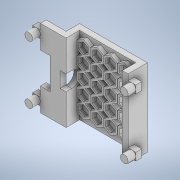
# Autodesk Inventor part: f2_grip
Saved by Autodesk Inventor 2020 (Build 240168000, 168)
## iProperties
Created: 2019-10-20
Part Number: f2_grip
Material: Generic
Document SubType Name: Modeling
Designer: ayad493
Density: 1 g/cm^3
Appearance: Default
Author: ayad493
Autodesk Inventor part; units mm, degrees
ref_plane "YZ Plane" through (0, 0, 0) normal (1, 0, 0) x (0, 1, 0)
ref_plane "XZ Plane" through (0, 0, 0) normal (0, 1, 0) x (-1, 0, 0)
ref_plane "XY Plane" through (0, 0, 0) normal (0, 0, 1) x (1, 0, 0)
sketch "Sketch1" plane through (0, 0, 0) normal (0, 0, 1) x (1, 0, 0)
  line L0 (0, 0) -> (16, 0)
  line L1 (16, 0) -> (16, -20)
  line L2 (16, -20) -> (0, -20)
  line L3 (0, -20) -> (0, 0)
  line L4 (16, 0) -> (14.5, 0)
  line L5 (14.5, 0) -> (14.5, -20)
  line L6 (16, 0) -> (16, -1.5)
  line L7 (16, -1.5) -> (18, -1.5)
  line L8 (18, -1.5) -> (18, -3.5)
  line L9 (18, -3.5) -> (16, -3.5)
  line L10 (16, -3.5) -> (16, -1.5)
  line L11 (16, -20) -> (16, -18.5)
  line L12 (16, -18.5) -> (18, -18.5)
  line L13 (18, -18.5) -> (18, -16.5)
  line L14 (18, -16.5) -> (16, -16.5)
  line L15 (16, -16.5) -> (16, -18.5)
  line L16 (18, -2.5) -> (-8.623, -2.5)
  line L17 (-8.623, -2.5) -> (-8.623, -1.5)
  line L18 (-8.623, -1.5) -> (-6.623, -1.5)
  line L19 (-6.623, -1.5) -> (-6.623, -3.5)
  line L20 (-6.623, -3.5) -> (-8.623, -3.5)
  line L21 (-8.623, -3.5) -> (-8.623, -1.5)
  line L22 (0, 0) -> (-6.623, 0)
  line L23 (-6.623, 0) -> (-6.623, -20)
  line L24 (-6.623, -20) -> (0, -20)
  line L25 (18, -17.5) -> (-6.623, -17.5)
  line L26 (-6.623, -17.5) -> (-6.623, -16.5)
  line L27 (-6.623, -16.5) -> (-8.623, -16.5)
  line L28 (-8.623, -16.5) -> (-8.623, -18.5)
  line L29 (-8.623, -18.5) -> (-6.623, -18.5)
  line L30 (-6.623, -18.5) -> (-6.623, -16.5)
  dimension "d0" = 16
  dimension "d1" = 20
  dimension "d2" = 90
  dimension "d3" = 1.5
  dimension "d4" = 1.5
  dimension "d5" = 2
  dimension "d6" = 2
  dimension "d7" = 1.5
  dimension "d8" = 2
  dimension "d9" = 2
  dimension "d10" = 26.623
  dimension "d11" = 2
  dimension "d12" = 1
  dimension "d13" = 2
  constraints: 62 end point, 9 perpendicular, 8 parallel, 7 horizontal, 7 point on line, 2 midpoint, 1 collinear, 1 vertical
  measures "d0" distance of L0.start L0.end
  measures "d1" distance of L0.end L1.end
  measures "d2" angle of L0 L1
  measures "d3" distance of L0.end L4.end
  measures "d4" distance of L0.end L6.end
  measures "d5" distance of L8.end L9.end
  measures "d6" distance of L7.end L8.end
  measures "d7" distance of L1.end L11.end
  measures "d8" distance of L14.end L13.end
  measures "d9" distance of L12.end L13.end
  measures "d10" distance of L16.start L16.end
  measures "d11" distance of L19.end L20.end
  measures "d12" distance of L25.end L26.end
  measures "d13" distance of L29.end L28.end
extrude "Extrusion1" add sketch "Sketch1" along normal blind 1.5
sketch "Sketch2" plane through (0, 0, 1.5) normal (0, 0, 1) x (1, 0, 0)
  line L0 (-8.623, -1.5) -> (-8.623, -3.5) projected
  line L1 (-8.623, -3.5) -> (-6.623, -3.5) projected
  line L2 (-8.623, -1.5) -> (-6.623, -3.5)
  line L3 (18, -3.5) -> (18, -1.5) projected
  line L4 (16, -16.5) -> (16, -3.5) projected
  line L5 (18, -1.5) -> (16, -3.5)
  line L6 (-6.623, -16.5) -> (-8.623, -16.5) projected
  line L7 (-6.623, -18.5) -> (-6.623, -20) projected
  line L8 (-8.623, -16.5) -> (-6.623, -18.5)
  line L9 (16, -18.5) -> (18, -18.5) projected
  line L10 (18, -16.5) -> (16, -16.5) projected
  line L11 (16, -18.5) -> (18, -16.5)
  circle A0 centre (-7.623, -2.5) radius 1
  circle A1 centre (17, -2.5) radius 1
  circle A2 centre (17, -17.5) radius 1
  circle A3 centre (-7.623, -17.5) radius 1
  point P0 (0, 0)
  constraints: 8 end point, 4 centre point, 4 midpoint
extrude "Extrusion2" add sketch "Sketch2" along normal blind 2 contours A0 L2 | A0 L2 | A1 L5 | A2 L11 | L5 A1 | A2 L11 | A3 L8 | L8 A3
sketch "Sketch3" plane through (0, 0, 0) normal (0, 0, -1) x (-1, 0, 0)
  line L0 (6.623, -18.5) -> (6.623, -20) projected
  line L1 (6.623, -20) -> (0, -20)
  line L2 (0, -20) -> (0, 0)
  line L3 (0, 0) -> (6.623, 0)
  line L4 (6.623, 0) -> (6.623, -20)
  line L5 (6.623, -20) -> (-16, -20) projected
  line L6 (-16, 0) -> (6.623, 0) projected
  line L7 (-16, -20) -> (-14.5, -20)
  line L8 (-14.5, -20) -> (-14.5, 0)
  line L9 (-14.5, 0) -> (-16, 0)
  line L10 (-16, 0) -> (-16, -20)
  line L11 (6.623, -20) -> (-16, -20)
  line L12 (-16, -20) -> (-16, -18.5)
  line L13 (-16, -18.5) -> (6.623, -18.5)
  line L14 (6.623, -18.5) -> (6.623, -20)
  line L15 (-16, 0) -> (6.623, 0)
  line L16 (6.623, 0) -> (6.623, -1.5)
  line L17 (6.623, -1.5) -> (-16, -1.5)
  line L18 (-16, -1.5) -> (-16, 0)
  point P0 (0, -1.5)
  point P1 (0, -18.5)
  point P2 (-14.5, -18.5)
  point P3 (-14.5, -1.5)
  dimension "d18" = 1.5
  constraints: 32 end point, 8 parallel, 4 horizontal, 4 perpendicular, 1 point on line
  measures "d18" distance of L9.end L8.end
extrude "Extrusion3" add sketch "Sketch3" along normal blind 5 contours L13 L2 L17 L4 | L0 L1 L2 L13 | L17 L2 L3 L4 | L2 L5 L8 L13 | L17 L8 L6 L2 | L13 L10 L17 L8 | L8 L5 L10 L13 | L17 L10 L6 L8
sketch "Sketch4" plane through (0, 0, 0) normal (0, 0, -1) x (-1, 0, 0)
  line L0 (-14.5, -18.5) -> (0, -18.5) projected
  line L1 (-14.5, -18.5) -> (-14.5, -1.5) projected
  line L2 (0, -18.5) -> (-14.5, -18.5)
  line L3 (-14.5, -18.5) -> (-14.5, -1.5)
  line L4 (-14.5, -1.5) -> (0, -1.5)
  line L5 (0, -1.5) -> (0, -18.5)
  point P0 (0, 0)
  constraints: 8 end point, 2 parallel, 1 horizontal, 1 perpendicular
extrude "Extrusion4" cut sketch "Sketch4" against normal through all
sketch "Sketch5" plane through (-6.623, 0, 1.5) normal (0, 1, 0) x (1, 0, 0)
  line L0 (22.623, 6.5) -> (22.623, 0) projected
  line L1 (0, 6.5) -> (22.623, 6.5)
  line L2 (22.623, 6.5) -> (22.623, 5)
  line L3 (22.623, 5) -> (0, 5)
  line L4 (0, 5) -> (0, 6.5)
  point P0 (6.623, 1.5)
  dimension "d23" = 1.5
  constraints: 8 end point, 2 parallel, 1 horizontal, 1 perpendicular, 1 point on line
  measures "d23" distance of L1.end L2.end
extrude "Extrusion5" add sketch "Sketch5" against normal up to surface (20 mm away)
sketch "Sketch7" plane through (-6.623, -20, 1.5) normal (0, -1, 0) x (1, 0, 0)
  line L0 (21.123, 0) -> (6.623, 0) projected
  line L1 (22.623, -6.5) -> (0, -6.5) projected
  line L2 (6.623, 0) -> (5.123, 0)
  line L3 (5.123, 0) -> (5.123, -6.5)
  line L4 (5.123, -6.5) -> (6.623, -6.5)
  line L5 (6.623, -6.5) -> (6.623, 0)
  line L6 (0, -6.5) -> (0, 0) projected
  line L7 (5.123, -6.5) -> (0, -6.5)
  line L8 (0, -6.5) -> (0, -1.5)
  line L9 (0, -1.5) -> (5.123, -1.5)
  line L10 (5.123, -1.5) -> (5.123, -6.5)
  point P0 (6.623, -1.5)
  dimension "d31" = 1.5
  constraints: 16 end point, 4 parallel, 2 horizontal, 2 perpendicular, 2 point on line
  measures "d31" distance of L4.end L3.end
extrude "Extrusion7" cut sketch "Sketch7" against normal through all contours L1 L6 L9 L3
sketch "Sketch8" plane through (-6.623, -20, 1.5) normal (0, -1, 0) x (1, 0, 0)
  line L0 (22.623, -6.5) -> (22.623, 0) projected
  line L1 (5.123, -1.5) -> (5.123, -6.5) projected
  line L2 (22.623, -6.5) -> (5.123, -6.5)
  line L3 (5.123, -6.5) -> (5.123, -4.9793)
  line L4 (5.123, -4.9793) -> (22.623, -4.9793)
  line L5 (22.623, -4.9793) -> (22.623, -6.5)
  point P0 (6.623, -1.5)
  constraints: 8 end point, 2 parallel, 1 horizontal, 1 perpendicular, 1 point on line
extrude "Extrusion8" cut sketch "Sketch8" against normal through all
sketch "Sketch9" plane through (-6.623, -20, 1.5) normal (0, -1, 0) x (1, 0, 0)
  line L0 (5.123, -4.9793) -> (22.623, -4.9793) projected
  line L1 (5.123, -1.5) -> (5.123, -4.9793) projected
  line L2 (22.623, -4.9793) -> (5.123, -4.9793)
  line L3 (5.123, -4.9793) -> (5.123, -3.4793)
  line L4 (5.123, -3.4793) -> (22.623, -3.4793)
  line L5 (22.623, -3.4793) -> (22.623, -4.9793)
  point P0 (6.623, -1.5)
  dimension "d36" = 1.5
  constraints: 8 end point, 2 parallel, 1 horizontal, 1 perpendicular, 1 point on line
  measures "d36" distance of L2.end L3.end
extrude "Extrusion9" add sketch "Sketch9" against normal up to surface (20 mm away)
sketch "Sketch10" plane through (-6.623, -16.5, 0) normal (-1, 0, 0) x (0, 0, 1)
  line L0 (0, 13) -> (0, 0) projected
  line L1 (1.5, 0) -> (1.5, 13) projected
  line L2 (0, 6.5) -> (1.5, 6.5)
  line L3 (1.5, 6.5) -> (1.5, 2.5)
  line L4 (1.5, 2.5) -> (0, 2.5)
  line L5 (0, 2.5) -> (0, 6.5)
  line L6 (1.5, 6.5) -> (0, 6.5)
  line L7 (0, 6.5) -> (0, 10.5)
  line L8 (0, 10.5) -> (1.5, 10.5)
  line L9 (1.5, 10.5) -> (1.5, 6.5)
  point P0 (0, 16.5)
  point P1 (0, 2.5)
  dimension "d39" = 4
  dimension "d40" = 4
  constraints: 16 end point, 4 parallel, 2 horizontal, 2 perpendicular, 2 point on line, 1 midpoint
  measures "d39" distance of L2.end L3.end
  measures "d40" distance of L6.end L7.end
extrude "Extrusion10" cut sketch "Sketch10" against normal up to surface (5.123 mm away)
sketch "Sketch12" plane through (0, -18.5, -1.9793) normal (0, 0, 1) x (1, 0, 0)
  line L0 (14.5, 0) -> (0, 0) projected
  line L1 (14.5, 17) -> (14.5, 0) projected
  line L2 (14.5, 0) -> (14.5, 4)
  line L3 (12.5, 0) -> (10.7679, 1)
  line L4 (10.7679, 1) -> (10.7679, 3)
  line L5 (10.7679, 3) -> (12.5, 4)
  line L6 (12.5, 4) -> (14.2321, 3)
  line L7 (14.2321, 3) -> (14.2321, 1)
  line L8 (14.2321, 1) -> (12.5, 0)
  line L9 (11.2679, 1.2887) -> (12.5, 0.5774)
  line L10 (12.5, 0.5774) -> (13.7321, 1.2887)
  line L11 (13.7321, 1.2887) -> (13.7321, 2.7113)
  line L12 (13.7321, 2.7113) -> (12.5, 3.4226)
  line L13 (12.5, 3.4226) -> (11.2679, 2.7113)
  line L14 (11.2679, 2.7113) -> (11.2679, 1.2887)
  point P0 (0, 18.5)
  point P1 (12.6339, 0.5)
  point P2 (12.5, 2)
  dimension "d55" = 4
  dimension "d56" = 0.5
  constraints: 26 end point, 1 point on line, 18 other
  measures "d55" distance of L0.start L2.end
  measures "d56" distance between parallel lines of L3 L9
extrude "Extrusion12" add sketch "Sketch12" along normal blind 1
sketch "Sketch11" plane through (-1.5, -20, -3.4793) normal (-1, 0, 0) x (0, 0, 1)
  line L0 (0, 0) -> (0, 20) projected
  line L1 (4.9793, 14) -> (4.9793, 6) projected
  line L2 (4.9793, 10) -> (3.4793, 10)
  circle A0 centre (3.4793, 10) radius 2
  point P0 (3.4793, 20)
  point P1 (4.9793, 11.3229)
  point P2 (4.9793, 8.6771)
  dimension "d43" = 1.5
  dimension "d44" = 4
  constraints: 2 end point, 1 centre point, 1 coincident, 1 horizontal, 1 midpoint
  measures "d43" distance of L2.start L2.end
  measures "d44" diameter of A0
extrude "Extrusion11" cut sketch "Sketch11" against normal blind 2 contours L1 A0 picked at (2.6654, 10.1597)
sketch "Sketch13" plane through (-6.623, -20, 1.5) normal (0, -1, 0) x (1, 0, 0)
  line L0 (6.623, 0) -> (6.623, -3.4793) projected
  line L1 (21.1544, -3.4793) -> (6.623, -3.4793)
  line L2 (6.623, -3.4793) -> (6.623, 0)
  line L3 (6.623, 0) -> (21.1544, 0)
  line L4 (0, 0) -> (22.623, 0) projected
  line L5 (21.123, -3.4793) -> (21.123, 0) projected
  line L6 (21.123, -3.4793) -> (21.123, 0)
  point P0 (6.623, -1.5)
  constraints: 8 end point, 2 collinear, 1 horizontal, 1 point on line
extrude "Extrusion13" cut sketch "Sketch13" against normal blind 1.5
sketch "Sketch14" plane through (-6.623, 0, 1.5) normal (0, 1, 0) x (1, 0, 0)
  line L0 (21.123, 0) -> (21.123, 3.4793) projected
  line L1 (21.123, 3.4793) -> (6.623, 3.4793) projected
  line L2 (21.123, 0) -> (6.623, 0)
  line L3 (6.623, 0) -> (6.623, 3.4793)
  line L4 (6.623, 3.4793) -> (21.123, 3.4793)
  line L5 (21.123, 3.4793) -> (21.123, 0)
  point P0 (6.623, 1.5)
  constraints: 8 end point, 2 parallel, 1 horizontal, 1 perpendicular
extrude "Extrusion14" cut sketch "Sketch14" against normal blind 1.5
pattern_linear "Rectangular Pattern1" count 4 spacing 3.5 along (-1, 0, 0) count 5 spacing 3.5 along (0, 1, 0) of "Extrusion12"
sketch "Sketch15" plane through (-6.623, 0, 1.5) normal (0, 1, 0) x (1, 0, 0)
  line L0 (6.623, 3.4793) -> (6.623, 0) projected
  line L1 (0, 1.5) -> (5.123, 1.5) projected
  line L2 (6.623, 0) -> (2.5615, 0)
  line L3 (2.5615, 0) -> (2.5615, 1.5)
  line L4 (2.5615, 1.5) -> (6.623, 1.5)
  line L5 (6.623, 1.5) -> (6.623, 0)
  constraints: 8 end point, 2 parallel, 1 horizontal, 1 midpoint, 1 perpendicular
extrude "Extrusion15" add sketch "Sketch15" against normal up to surface (20 mm away)
sketch "Sketch16" plane through (0, 0, 0) normal (0, 0, -1) x (-1, 0, 0)
  line L0 (1.5, -12) -> (0, -12) projected
  line L1 (1.5, 0) -> (1.5, -20) projected
  line L2 (0, -12) -> (1.5, -12)
  line L3 (1.5, -12) -> (1.5, -7.9843)
  line L4 (1.5, -7.9843) -> (0, -7.9843)
  line L5 (0, -7.9843) -> (0, -12)
  point P0 (0, 0)
  constraints: 8 end point, 2 parallel, 1 horizontal, 1 perpendicular, 1 point on line
extrude "Extrusion16" cut sketch "Sketch16" against normal blind 1.5
body "Solid1"
